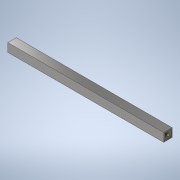
# Autodesk Inventor part: Part2
Saved by Autodesk Inventor 2020 (Build 240168000, 168)
## iProperties
Created: 2020-12-25
Part Number: Part2
Material: Steel, Mild
Document SubType Name: Modeling
Designer: Vikki
Mass: 317.062 g
Surface Area: 885.708 cm^2
Volume: 40.39 cm^3
Density: 7.85 g/cm^3
Appearance: Semi-Polished
Author: Vikki
Autodesk Inventor part; units mm, degrees
ref_plane "YZ Plane" through (0, 0, 0) normal (1, 0, 0) x (0, 1, 0)
ref_plane "XZ Plane" through (0, 0, 0) normal (0, 1, 0) x (-1, 0, 0)
ref_plane "XY Plane" through (0, 0, 0) normal (0, 0, 1) x (1, 0, 0)
sketch "Sketch1" plane through (0, 0, 0) normal (1, 0, 0) x (0, 1, 0)
  line L0 (-9.525, 9.525) -> (9.525, 9.525)
  line L1 (9.525, 9.525) -> (9.525, -9.525)
  line L2 (9.525, -9.525) -> (-9.525, -9.525)
  line L3 (-9.525, -9.525) -> (-9.525, 9.525)
  line L4 (-9.525, 9.525) -> (9.525, -9.525) construction
  line L5 (9.525, 9.525) -> (-9.525, -9.525) construction
  line L6 (-6.35, 6.35) -> (6.35, 6.35)
  line L7 (6.35, 6.35) -> (6.35, -6.35)
  line L8 (6.35, -6.35) -> (-6.35, -6.35)
  line L9 (-6.35, -6.35) -> (-6.35, 6.35)
  line L10 (-6.35, 6.35) -> (6.35, -6.35) construction
  line L11 (6.35, 6.35) -> (-6.35, -6.35) construction
  line L12 (-7.15, -7.15) -> (7.15, -7.15)
  line L13 (7.15, -7.15) -> (7.15, 7.15)
  line L14 (7.15, 7.15) -> (-7.15, 7.15)
  line L15 (-7.15, 7.15) -> (-7.15, -7.15)
  line L16 (-8.525, -8.525) -> (8.525, -8.525)
  line L17 (8.525, -8.525) -> (8.525, 8.525)
  line L18 (8.525, 8.525) -> (-8.525, 8.525)
  line L19 (-8.525, 8.525) -> (-8.525, -8.525)
  point P0 (0, 0)
  dimension "d0" = 19.05
  dimension "d1" = 12.7
  dimension "d2" = 0.8
  dimension "d3" = 1
  constraints: 40 end point, 8 parallel, 6 perpendicular, 4 midpoint, 2 horizontal, 6 other
  measures "d0" distance of L0.end L1.end
  measures "d1" distance of L8.end L6.start
  measures "d2" distance between parallel lines of L12 L8
  measures "d3" distance between parallel lines of L2 L16
extrude "Extrusion1" add sketch "Sketch1" along normal blind 350
sketch "Sketch2" plane through (350, 0, 0) normal (1, 0, 0) x (0, 0, -1)
  point P0 (0, 0)
sketch "Sketch3" plane through (350, 0, 0) normal (1, 0, 0) x (0, 0, -1)
  circle A0 centre (0, 0) radius 15.1328
  constraints: 1 centre point, 1 coincident
surface extrude "ExtrusionSrf1" sketch "Sketch3" against normal blind 350 shown no curves A0
body "Solid1"
body "Srf1"
